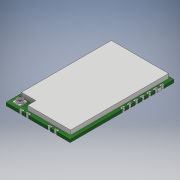
# Autodesk Inventor part: E22-400T30XX
Saved by Autodesk Inventor 2018 (Build 220112000, 112)
## iProperties
Created: 2022-01-24
Part Number: E22-400T30XX
Material: Типовые
Document SubType Name: Modeling
Designer: Nurekengoi
Density: 1 g/cm^3
Appearance: По умолчанию
Author: Nurekengoi
Autodesk Inventor part; units mm, degrees
ref_plane "YZ Plane" through (0, 0, 0) normal (1, 0, 0) x (0, 1, 0)
ref_plane "XZ Plane" through (0, 0, 0) normal (0, 1, 0) x (-1, 0, 0)
ref_plane "XY Plane" through (0, 0, 0) normal (0, 0, 1) x (1, 0, 0)
sketch "Эскиз1" plane through (0, 0, 0) normal (0, 0, 1) x (1, 0, 0)
  line L0 (-12.5, 20.25) -> (12.5, 20.25)
  line L1 (12.5, 20.25) -> (12.5, -20.25)
  line L2 (12.5, -20.25) -> (-12.5, -20.25)
  line L3 (-12.5, -20.25) -> (-12.5, 20.25)
  circle A0 centre (12.5, 15.87) radius 0.45
  circle A1 centre (12.5, 13.33) radius 0.45
  circle A2 centre (12.5, 10.79) radius 0.45
  circle A3 centre (12.5, 8.25) radius 0.45
  circle A4 centre (12.5, 5.71) radius 0.45
  circle A5 centre (12.5, 3.17) radius 0.45
  circle A6 centre (12.5, 0.63) radius 0.45
  line L4 (0, 0) -> (0, 16.5356)
  circle A7 centre (-12.5, 15.87) radius 0.45
  circle A8 centre (-12.5, 13.33) radius 0.45
  circle A9 centre (-12.5, 10.79) radius 0.45
  circle A10 centre (-12.5, 8.25) radius 0.45
  circle A11 centre (-12.5, 5.71) radius 0.45
  circle A12 centre (-12.5, 3.17) radius 0.45
  circle A13 centre (-12.5, 0.63) radius 0.45
  circle A14 centre (6.77, -20.25) radius 0.45
  circle A15 centre (4.23, -20.25) radius 0.45
  circle A16 centre (-6.77, -20.25) radius 0.45
  circle A17 centre (-4.23, -20.25) radius 0.45
  point P0 (0, 20.25)
  point P1 (12.5, 0)
  dimension "d0" = 25
  dimension "d1" = 40.5
  dimension "d2" = 0.9
  dimension "d3" = 4.38
  dimension "d6" = 2.54
  dimension "d11" = 0.9
  dimension "d12" = 5.73
  dimension "d15" = 2.54
  constraints: 18 centre point, 10 end point, 9 symmetric about line, 2 horizontal, 2 midpoint, 2 parallel, 2 point on line, 2 vertical, 1 horizontal alignment, 1 perpendicular, 1 vertical alignment, 23 other
  measures "d0" distance of L1.end L2.end
  measures "d1" distance of L0.end L1.end
  measures "d2" diameter of A0
  measures "d3" distance from line of L0 A0.centre
  measures "d6" distance of A0.centre A1.centre
  measures "d11" diameter of A14
  measures "d12" distance from line of L1 A14.centre
  measures "d15" distance of A14.centre A15.centre
extrude "Выдавливание1" add sketch "Эскиз1" along normal blind 1.2 contours L0 L1 A0 A1 A2 A3 A4 A5 A6 L2 A14 A15 A17 A16 L3 A13 A12 A11 A10 A9 A8 A7 | A7 L3 | L1 A0 | A8 L3 | L1 A1 | A9 L3 | L1 A2 | A10 L3 | L1 A3 | A11 L3 | L1 A4 | A12 L3 | L1 A5 | A13 L3 | L1 A6 | A16 L2 | L2 A14 | A17 L2 | L2 A15 picked at (-12.2843, 15.9746) picked at (12.3511, 15.8519) picked at (-12.3698, 13.18) picked at (12.3511, 13.3119) picked at (-12.4349, 10.9251) picked at (12.3511, 10.7719) picked at (-12.4015, 8.3889) picked at (12.3511, 8.2319) picked at (-12.2526, 5.8035) picked at (12.3511, 5.6919) picked at (-12.2526, 3.2635) picked at (12.3511, 3.1519) picked at (-12.2526, 0.7235) picked at (12.3511, 0.6119) picked at (-6.7519, -20.1011) picked at (6.7881, -20.1011) picked at (-4.2119, -20.1011) picked at (4.2481, -20.1011)
sketch "Эскиз4" plane through (0, 0, 1.2) normal (0, 0, 1) x (1, 0, 0)
  line L0 (-12.5, 20.25) -> (-12.5, -20.25) projected
  line L1 (-12.5, 16.62) -> (-11.75, 16.62)
  line L2 (-11.75, 16.62) -> (-11.75, 15.12)
  line L3 (-11.75, 15.12) -> (-12.5, 15.12)
  line L4 (-12.5, 15.12) -> (-12.5, 16.62)
  line L5 (12.5, 20.25) -> (-12.5, 20.25) projected
  line L6 (-12.5, 14.08) -> (-11.75, 14.08)
  line L7 (-11.75, 14.08) -> (-11.75, 12.58)
  line L8 (-11.75, 12.58) -> (-12.5, 12.58)
  line L9 (-12.5, 12.58) -> (-12.5, 14.08)
  line L10 (-12.5, 11.54) -> (-11.75, 11.54)
  line L11 (-11.75, 11.54) -> (-11.75, 10.04)
  line L12 (-11.75, 10.04) -> (-12.5, 10.04)
  line L13 (-12.5, 10.04) -> (-12.5, 11.54)
  line L14 (-12.5, 9) -> (-11.75, 9)
  line L15 (-11.75, 9) -> (-11.75, 7.5)
  line L16 (-11.75, 7.5) -> (-12.5, 7.5)
  line L17 (-12.5, 7.5) -> (-12.5, 9)
  line L18 (-12.5, 6.46) -> (-11.75, 6.46)
  line L19 (-11.75, 6.46) -> (-11.75, 4.96)
  line L20 (-11.75, 4.96) -> (-12.5, 4.96)
  line L21 (-12.5, 4.96) -> (-12.5, 6.46)
  line L22 (-12.5, 3.92) -> (-11.75, 3.92)
  line L23 (-11.75, 3.92) -> (-11.75, 2.42)
  line L24 (-11.75, 2.42) -> (-12.5, 2.42)
  line L25 (-12.5, 2.42) -> (-12.5, 3.92)
  line L26 (-12.5, 1.38) -> (-11.75, 1.38)
  line L27 (-11.75, 1.38) -> (-11.75, -0.12)
  line L28 (-11.75, -0.12) -> (-12.5, -0.12)
  line L29 (-12.5, -0.12) -> (-12.5, 1.38)
  line L30 (0, 0) -> (0, 23.8656)
  line L31 (12.5, 16.62) -> (11.75, 16.62)
  line L32 (11.75, 16.62) -> (11.75, 15.12)
  line L33 (11.75, 15.12) -> (12.5, 15.12)
  line L34 (12.5, 15.12) -> (12.5, 16.62)
  line L35 (12.5, 14.08) -> (11.75, 14.08)
  line L36 (11.75, 14.08) -> (11.75, 12.58)
  line L37 (11.75, 12.58) -> (12.5, 12.58)
  line L38 (12.5, 12.58) -> (12.5, 14.08)
  line L39 (12.5, 11.54) -> (11.75, 11.54)
  line L40 (11.75, 11.54) -> (11.75, 10.04)
  line L41 (11.75, 10.04) -> (12.5, 10.04)
  line L42 (12.5, 10.04) -> (12.5, 11.54)
  line L43 (12.5, 9) -> (11.75, 9)
  line L44 (11.75, 9) -> (11.75, 7.5)
  line L45 (11.75, 7.5) -> (12.5, 7.5)
  line L46 (12.5, 7.5) -> (12.5, 9)
  line L47 (12.5, 6.46) -> (11.75, 6.46)
  line L48 (11.75, 6.46) -> (11.75, 4.96)
  line L49 (11.75, 4.96) -> (12.5, 4.96)
  line L50 (12.5, 4.96) -> (12.5, 6.46)
  line L51 (12.5, 3.92) -> (11.75, 3.92)
  line L52 (11.75, 3.92) -> (11.75, 2.42)
  line L53 (11.75, 2.42) -> (12.5, 2.42)
  line L54 (12.5, 2.42) -> (12.5, 3.92)
  line L55 (12.5, 1.38) -> (11.75, 1.38)
  line L56 (11.75, 1.38) -> (11.75, -0.12)
  line L57 (11.75, -0.12) -> (12.5, -0.12)
  line L58 (12.5, -0.12) -> (12.5, 1.38)
  line L59 (-12.5, -20.25) -> (12.5, -20.25) projected
  line L60 (-7.52, -20.25) -> (-6.02, -20.25)
  line L61 (-6.02, -20.25) -> (-6.02, -19.5)
  line L62 (-6.02, -19.5) -> (-7.52, -19.5)
  line L63 (-7.52, -19.5) -> (-7.52, -20.25)
  line L64 (-3.48, -19.5) -> (-4.98, -19.5)
  line L65 (-4.98, -19.5) -> (-4.98, -20.25)
  line L66 (-3.48, -20.25) -> (-3.48, -19.5)
  line L67 (-4.98, -20.25) -> (-3.48, -20.25)
  line L68 (7.52, -20.25) -> (6.02, -20.25)
  line L69 (6.02, -20.25) -> (6.02, -19.5)
  line L70 (6.02, -19.5) -> (7.52, -19.5)
  line L71 (7.52, -19.5) -> (7.52, -20.25)
  line L72 (3.48, -19.5) -> (4.98, -19.5)
  line L73 (4.98, -19.5) -> (4.98, -20.25)
  line L74 (3.48, -20.25) -> (3.48, -19.5)
  line L75 (4.98, -20.25) -> (3.48, -20.25)
  point P0 (-11.75, 15.87)
  point P1 (-11.75, 13.33)
  point P2 (-11.75, 10.79)
  point P3 (-11.75, 8.25)
  point P4 (-11.75, 5.71)
  point P5 (-11.75, 3.17)
  point P6 (-11.75, 0.63)
  point P7 (11.75, 15.87)
  point P8 (11.75, 13.33)
  point P9 (11.75, 10.79)
  point P10 (11.75, 8.25)
  point P11 (11.75, 5.71)
  point P12 (11.75, 3.17)
  point P13 (11.75, 0.63)
  point P14 (-6.77, -19.5)
  point P15 (-4.23, -19.5)
  point P16 (6.77, -19.5)
  point P17 (4.23, -19.5)
  dimension "d77" = 0.75
  dimension "d78" = 1.5
  dimension "d79" = 4.38
  dimension "d82" = 2.54
  dimension "d87" = 1.5
  dimension "d88" = 0.75
  dimension "d89" = 5.73
  dimension "d92" = 2.54
  constraints: 146 end point, 45 symmetric about line, 4 parallel, 3 horizontal, 2 midpoint, 2 perpendicular, 2 point on line, 2 vertical, 63 other
  measures "d77" distance of L2.end L3.end
  measures "d78" distance of L1.end L2.end
  measures "d79" distance from line of L5 point (-11.75, 15.87)
  measures "d82" distance of L1.start L6.start
  measures "d87" distance of L62.end L61.end
  measures "d88" distance of L61.end L60.end
  measures "d89" distance from line of L0 point (-6.77, -19.5)
  measures "d92" distance of L62.end L64.end
extrude "Выдавливание4" add sketch "Эскиз4" along normal blind 0.1
sketch "Эскиз2" plane through (0, 0, 0) normal (0, 0, 1) x (1, 0, 0)
  line L0 (-12.5, 20.25) -> (12.5, 20.25)
  line L1 (12.5, 20.25) -> (12.5, -20.25)
  line L2 (12.5, -20.25) -> (-12.5, -20.25)
  line L3 (-12.5, -20.25) -> (-12.5, 20.25)
  circle A0 centre (12.5, 15.87) radius 0.45
  circle A1 centre (12.5, 13.33) radius 0.45
  circle A2 centre (12.5, 10.79) radius 0.45
  circle A3 centre (12.5, 8.25) radius 0.45
  circle A4 centre (12.5, 5.71) radius 0.45
  circle A5 centre (12.5, 3.17) radius 0.45
  circle A6 centre (12.5, 0.63) radius 0.45
  line L4 (0, 0) -> (0, 16.5356)
  circle A7 centre (-12.5, 15.87) radius 0.45
  circle A8 centre (-12.5, 13.33) radius 0.45
  circle A9 centre (-12.5, 10.79) radius 0.45
  circle A10 centre (-12.5, 8.25) radius 0.45
  circle A11 centre (-12.5, 5.71) radius 0.45
  circle A12 centre (-12.5, 3.17) radius 0.45
  circle A13 centre (-12.5, 0.63) radius 0.45
  circle A14 centre (6.77, -20.25) radius 0.45
  circle A15 centre (4.23, -20.25) radius 0.45
  circle A16 centre (-4.23, -20.25) radius 0.45
  circle A17 centre (-6.77, -20.25) radius 0.45
  point P0 (0, 20.25)
  point P1 (12.5, 0)
  dimension "d30" = 25
  dimension "d31" = 40.5
  dimension "d32" = 0.9
  dimension "d33" = 4.38
  dimension "d34" = 2.54
  dimension "d35" = 0.9
  dimension "d36" = 5.73
  dimension "d37" = 2.54
  constraints: 18 centre point, 10 end point, 9 symmetric about line, 2 horizontal, 2 midpoint, 2 parallel, 2 point on line, 2 vertical, 1 horizontal alignment, 1 perpendicular, 1 vertical alignment, 23 other
  measures "d30" distance of L1.end L2.end
  measures "d31" distance of L0.end L1.end
  measures "d32" diameter of A0
  measures "d33" distance from line of L0 A0.centre
  measures "d34" distance of A0.centre A1.centre
  measures "d35" diameter of A14
  measures "d36" distance from line of L1 A14.centre
  measures "d37" distance of A14.centre A15.centre
extrude "Выдавливание5" cut sketch "Эскиз2" along normal blind 2 contours A7 L3 | L3 A7 | A0 L1 | L1 A0 | A8 L3 | L3 A8 | A1 L1 | L1 A1 | A9 L3 | L3 A9 | A2 L1 | L1 A2 | A10 L3 | L3 A10 | A3 L1 | L1 A3 | A11 L3 | L3 A11 | A4 L1 | L1 A4 | A12 L3 | L3 A12 | A5 L1 | L1 A5 | A13 L3 | L3 A13 | A6 L1 | L1 A6 | A17 L2 | L2 A17 | A14 L2 | L2 A14 | A16 L2 | L2 A16 | A15 L2 | L2 A15
sketch "Эскиз5" plane through (0, 0, 1.2) normal (0, 0, 1) x (1, 0, 0)
  line L0 (12.4911, 20.0783) -> (12.4911, -20.2296) construction
  line L1 (12.4911, -20.2296) -> (-12.3051, -20.2296) construction
  line L2 (-12.3051, -20.2296) -> (-12.3051, 20.0783) construction
  line L3 (-12.3051, 20.0783) -> (12.4911, 20.0783) construction
  line L4 (-11.1629, 19.4744) -> (11.229, 19.4744)
  line L5 (11.229, 19.4744) -> (11.229, -18.8086)
  line L6 (11.229, -18.8086) -> (-5.546, -18.8086)
  line L7 (-5.546, -18.8086) -> (-5.546, -15.6466)
  line L8 (-5.546, -15.6466) -> (-11.1629, -15.6466)
  line L9 (-11.1629, -15.6466) -> (-11.1629, 19.4744)
  circle A0 centre (-9.6707, -17.6676) radius 1.2359
  circle A1 centre (-9.6707, -17.6676) radius 1.0068
  point P0 (0, 0)
  constraints: 12 end point, 5 perpendicular, 2 centre point, 1 coincident, 1 parallel, 2 other
extrude "Выдавливание6" add sketch "Эскиз5" along normal blind 1.7
sketch "Эскиз6" plane through (0, 0, 1.2) normal (0, 0, 1) x (1, 0, 0)
  line L0 (-8.1707, -16.1676) -> (-11.1707, -16.1676)
  line L1 (-11.1707, -16.1676) -> (-11.1707, -19.1676)
  line L2 (-11.1707, -19.1676) -> (-8.1707, -19.1676)
  line L3 (-8.1707, -19.1676) -> (-8.1707, -16.1676)
  circle A0 centre (-9.6707, -17.6676) radius 1.0068 projected
  point P0 (0, 0)
  point P1 (-8.1707, -17.6676)
  point P2 (-9.6707, -19.1676)
  dimension "d158" = 0
  dimension "d159" = 3
  dimension "d160" = 0
  dimension "d161" = 3
  constraints: 8 end point, 2 midpoint, 2 parallel, 1 horizontal, 1 perpendicular
  measures "d158" vertical distance of A0.centre point (-8.171, -17.668)
  measures "d159" distance between parallel lines of L1 L3
  measures "d160" horizontal distance of A0.centre point (-9.671, -19.168)
  measures "d161" distance of L0.end L1.end
extrude "Выдавливание7" add sketch "Эскиз6" along normal blind 0.4
sketch "Эскиз7" plane through (-9.6707, -17.6676, 2.9) normal (0, 0, 1) x (1, 0, 0)
  line L0 (-1.6698, -1.5644) -> (1.6741, -1.5644)
  line L1 (1.6741, -1.5644) -> (1.6741, 1.6132)
  line L2 (1.6741, 1.6132) -> (-1.6698, 1.6132)
  line L3 (-1.6698, 1.6132) -> (-1.6698, -1.5644)
  point P0 (9.6707, 17.6676)
  constraints: 8 end point, 2 parallel, 1 horizontal, 1 perpendicular
extrude "Выдавливание8" cut sketch "Эскиз7" against normal blind 0.5
